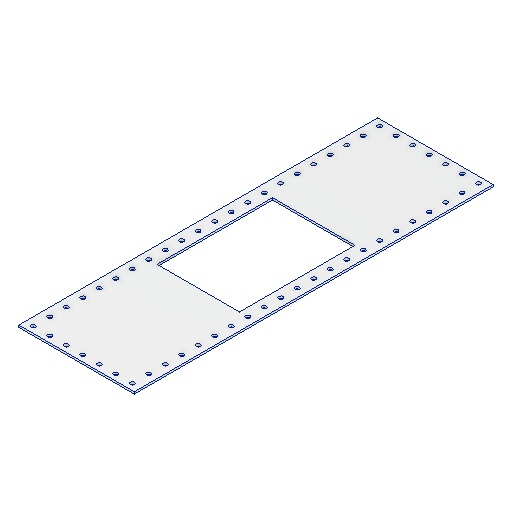
# Autodesk Inventor part: top plate 3
Saved by Autodesk Inventor 2022 (Build 260153000, 153)
## iProperties
Created: 2022-01-28
Part Number: top plate 3
Material: Aluminum 6061
Document SubType Name: Sheet Metal
Designer: 5126_Cad_5
Density: 2.7 g/cm^3
Sheet Metal Rule: Default
Appearance: Aluminum - Flat
Flat Pattern Width: 17.78 cm
Flat Pattern Length: 55.245 cm
Flat Pattern Area: 982.256 cm^2
Sheet Metal Width: 7.000 in
Sheet Metal Length: 21.750 in
Sheet Metal Area: 152.250 in^2
Author: 5126_Cad_5
Autodesk Inventor part; units mm, degrees
ref_plane "YZ Plane" through (0, 0, 0) normal (1, 0, 0) x (0, 1, 0)
ref_plane "XZ Plane" through (0, 0, 0) normal (0, 1, 0) x (-1, 0, 0)
ref_plane "XY Plane" through (0, 0, 0) normal (0, 0, 1) x (1, 0, 0)
sketch "Sketch1" plane through (0, 0, 0) normal (0, 1, 0) x (-1, 0, 0)
  line L0 (-88.9, -279.4) -> (88.9, -279.4)
  line L1 (88.9, -279.4) -> (88.9, 279.4)
  line L2 (88.9, 279.4) -> (-88.9, 279.4)
  line L3 (-88.9, 279.4) -> (-88.9, -279.4)
  line L4 (-88.9, -279.4) -> (88.9, 279.4) construction
  line L5 (88.9, -279.4) -> (-88.9, 279.4) construction
  point P0 (0, 0)
  dimension "d0" = 558.8
  dimension "d1" = 177.8
  measures "d0" distance of L1.end L0.end
  measures "d1" distance between parallel lines of L3 L1
extrude "Plate1" add sketch "Sketch1" along normal blind 3.175
sketch "Sketch2" plane through (0, 3.175, 0) normal (0, 1, 0) x (1, 0, 0)
  circle A0 centre (76.2, 266.7) radius 3.302
  line L0 (-88.9, 279.4) -> (88.9, 279.4) projected
  line L1 (88.9, 279.4) -> (88.9, -279.4) projected
  circle A1 centre (-68.6663, -258.1933) radius 3.302
  point P0 (0, 0)
  dimension "d3" = 6.604
  dimension "d4" = 12.7
  dimension "d5" = 12.7
  dimension "d14" = 6.604
  constraints: 2 centre point
  measures "d3" diameter of A0
  measures "d4" distance from line of L0 A0.centre
  measures "d5" distance from line of L1 A0.centre
  measures "d14" diameter of A1
extrude "Cut1" cut sketch "Sketch2" against normal blind 3.175 contours A0
pattern_linear "Rectangular Pattern1" count 22 spacing 25.4 along (0, 0, 1) of "Cut1"
pattern_linear "Rectangular Pattern2" count 6 spacing 25.4 along (-1, 0, 0) of "Cut1"
sketch "Sketch3" plane through (0, 3.175, 0) normal (0, 1, 0) x (1, 0, 0)
  circle A0 centre (-76.2, -266.7) radius 3.302
  line L0 (-88.9, -279.4) -> (-88.9, 279.4) projected
  line L1 (88.9, -279.4) -> (-88.9, -279.4) projected
  point P0 (0, 0)
  dimension "d15" = 6.604
  dimension "d16" = 12.7
  dimension "d17" = 12.7
  constraints: 1 centre point
  measures "d15" diameter of A0
  measures "d16" distance from line of L0 A0.centre
  measures "d17" distance from line of L1 A0.centre
extrude "Cut2" cut sketch "Sketch3" against normal blind 3.175
pattern_linear "Rectangular Pattern3" count 22 spacing 25.4 along (0, 0, -1) of "Cut2"
pattern_linear "Rectangular Pattern4" count 6 spacing 25.4 along (1, 0, 0) of "Cut2"
sketch "Sketch4" plane through (0, 3.175, 0) normal (0, 1, 0) x (1, 0, 0)
  line L0 (63.5, -88.9) -> (-63.5, -88.9)
  line L1 (-63.5, -88.9) -> (-63.5, 88.9)
  line L2 (-63.5, 88.9) -> (63.5, 88.9)
  line L3 (63.5, 88.9) -> (63.5, -88.9)
  line L4 (63.5, -88.9) -> (-63.5, 88.9) construction
  line L5 (-63.5, -88.9) -> (63.5, 88.9) construction
  point P0 (0, 0)
  dimension "d27" = 127
  dimension "d28" = 177.8
  constraints: 12 end point, 2 midpoint, 2 parallel, 1 horizontal, 1 perpendicular
  measures "d27" distance of L1.end L2.end
  measures "d28" distance of L0.end L1.end
extrude "Cut3" cut sketch "Sketch4" against normal blind 3.175
sketch "Sketch5" plane through (0, 3.175, 0) normal (0, 1, 0) x (1, 0, 0)
  line L0 (-88.9, 279.4) -> (-88.9, -279.4) projected
  line L1 (-88.9, -279.4) -> (88.9, -279.4)
  line L2 (88.9, -279.4) -> (88.9, -276.225)
  line L3 (88.9, -276.225) -> (-88.9, -276.225)
  line L4 (-88.9, -276.225) -> (-88.9, -279.4)
  line L5 (88.9, 279.4) -> (-88.9, 279.4) projected
  line L6 (-88.9, 279.4) -> (88.9, 279.4)
  line L7 (88.9, 279.4) -> (88.9, 276.225)
  line L8 (88.9, 276.225) -> (-88.9, 276.225)
  line L9 (-88.9, 276.225) -> (-88.9, 279.4)
  point P0 (0, 0)
  dimension "d31" = 177.8
  dimension "d32" = 3.175
  dimension "d33" = 177.8
  dimension "d34" = 3.175
  constraints: 16 end point, 4 parallel, 2 horizontal, 2 perpendicular
  measures "d31" distance of L3.end L2.end
  measures "d32" distance of L2.end L1.end
  measures "d33" distance of L7.end L8.end
  measures "d34" distance of L6.end L7.end
extrude "Cut4" cut sketch "Sketch5" against normal blind 3.175
equation "\"d6\" = Thickness"
equation "\"d18\" = Thickness"
equation "\"d29\" = Thickness"
equation "\"d35\" = Thickness"
equation "\"d2\" = Thickness"
equation "\"BendRadius\" = Thickness"
equation "\"BendReliefWidth\" = Thickness"
equation "\"BendReliefDepth\" = 0.5 * Thickness"
equation "\"CornerReliefSize\" = 4 * Thickness"
equation "\"MinimumRemnant\" = 2 * Thickness"
equation "\"TransitionRadius\" = BendRadius"
equation "\"JacobiRadiusSize\" = BendRadius"
equation "\"GapSize\" = Thickness"
equation "\"Thickness\" = 3.175"
body "Solid1"
